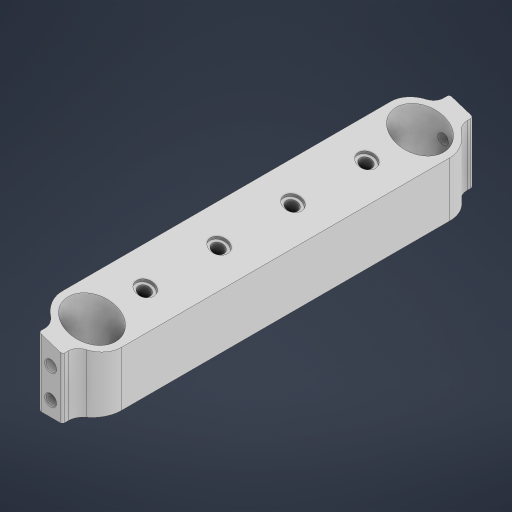
# Autodesk Inventor part: Leg_Battery_Connector
Saved by Autodesk Inventor 2023 (Build 270158000, 158)
## iProperties
Created: 2023-04-04
Part Number: Leg_Battery_Connector
Material: Generic
Document SubType Name: Modeling
Designer: dzw04
Density: 1 g/cm^3
Appearance: Default
Author: dzw04
Autodesk Inventor part; units mm, degrees
ref_plane "YZ Plane" through (0, 0, 0) normal (1, 0, 0) x (0, 1, 0)
ref_plane "XZ Plane" through (0, 0, 0) normal (0, 1, 0) x (-1, 0, 0)
ref_plane "XY Plane" through (0, 0, 0) normal (0, 0, 1) x (1, 0, 0)
sketch "Sketch1" plane through (0, 0, 0) normal (0, 1, 0) x (-1, 0, 0)
  line L0 (0, 0) -> (0, -55.5) construction
  circle A0 centre (0, -55.5) radius 8
  line L1 (0, 0) -> (10, 0) construction
  line L2 (0, 0) -> (-10, 0) construction
  line L3 (10, -55.5) -> (10, 0)
  line L4 (-10, -55.5) -> (-10, 0)
  line L5 (0, 0) -> (0, -12.5) construction
  line L6 (0, -12.5) -> (0, -37.5) construction
  line L7 (0, -65.5) -> (0, -69.5) construction
  line L8 (0, -69.5) -> (3.25, -69.5)
  line L9 (4, -68.75) -> (4, -67.5)
  line L10 (0, -69.5) -> (-3.25, -69.5)
  line L11 (-4, -68.75) -> (-4, -67.5)
  arc A1 (-10, -55.5) -> (-6, -63.5) centre (0, -55.5) ccw
  arc A2 (6, -63.5) -> (10, -55.5) centre (0, -55.5) ccw
  arc A3 (6, -63.5) -> (4, -67.5) centre (9, -67.5) ccw
  arc A4 (-4, -67.5) -> (-6, -63.5) centre (-9, -67.5) ccw
  arc A5 (-4, -68.75) -> (-3.25, -69.5) centre (-3.25, -68.75) ccw
  arc A6 (3.25, -69.5) -> (4, -68.75) centre (3.25, -68.75) ccw
  line L12 (0, 0) -> (0, 55.5) construction
  circle A7 centre (0, 55.5) radius 8
  line L13 (10, 55.5) -> (10, 0)
  line L14 (-10, 55.5) -> (-10, 0)
  line L15 (0, 0) -> (0, 12.5) construction
  line L16 (0, 12.5) -> (0, 37.5) construction
  line L17 (0, 65.5) -> (0, 69.5) construction
  line L18 (0, 69.5) -> (3.25, 69.5)
  line L19 (4, 68.75) -> (4, 67.5)
  line L20 (0, 69.5) -> (-3.25, 69.5)
  line L21 (-4, 68.75) -> (-4, 67.5)
  arc A8 (-6, 63.5) -> (-10, 55.5) centre (0, 55.5) ccw
  arc A9 (10, 55.5) -> (6, 63.5) centre (0, 55.5) ccw
  arc A10 (4, 67.5) -> (6, 63.5) centre (9, 67.5) ccw
  arc A11 (-6, 63.5) -> (-4, 67.5) centre (-9, 67.5) ccw
  arc A12 (-3.25, 69.5) -> (-4, 68.75) centre (-3.25, 68.75) ccw
  arc A13 (4, 68.75) -> (3.25, 69.5) centre (3.25, 68.75) ccw
  point P0 (4, -69.5)
  point P1 (4, -64.6652)
  point P2 (-4, -69.5)
  point P3 (-4, -64.6652)
  point P4 (4, 69.5)
  point P5 (4, 64.6652)
  point P6 (-4, 69.5)
  point P7 (-4, 64.6652)
  dimension "d0" = 55.5
  dimension "d1" = 16
  dimension "d3" = 10
  dimension "d4" = 10
  dimension "d6" = 12.5
  dimension "d7" = 25
  dimension "d10" = 4
  dimension "d11" = 4
  dimension "d12" = 4
  dimension "d13" = 5
  dimension "d14" = 0.75
  constraints: 44 end point, 28 point on circle, 25 symmetric about line, 16 point on line, 14 centre point, 10 tangent, 4 coincident, 4 horizontal, 2 equal radius, 2 perpendicular, 2 vertical, 7 other
  measures "d0" distance of L0.start L0.end
  measures "d1" diameter of A0
  measures "d3" distance of L0.start L1.end
  measures "d4" distance of L0.start L2.end
  measures "d6" distance of L0.start L5.end
  measures "d7" distance of L5.end L6.end
  measures "d10" distance of L7.start L7.end
  measures "d11" distance of L7.end point (4, -69.5)
  measures "d12" distance of L7.end point (-4, -69.5)
  measures "d13" radius of A3
  measures "d14" radius of A5
extrude "Extrusion1" add sketch "Sketch1" along normal blind 25
sketch "Sketch2" plane through (0, 0, 0) normal (0, 0, 1) x (1, 0, 0)
  line L0 (-10, 25) -> (10, 18.5016)
  line L1 (10, 0) -> (10, 25) projected
  line L2 (-10, 25) -> (11.0292, 25) construction
  line L3 (10, 18.5016) -> (10, 25)
  line L4 (10, 25) -> (-10, 25)
  point P0 (0, 0)
  dimension "d17" = 18
  constraints: 8 end point, 1 collinear, 1 equal length, 1 horizontal, 1 perpendicular, 1 point on line
  measures "d17" angle of L0 L2
extrude "Extrusion2" cut sketch "Sketch2" along normal through all both and the other way through all
sketch "Sketch3" plane through (10, 18.5016, 55.5) normal (0.309, 0.9511, 0) x (0.9511, -0.309, 0)
  ellipse E0 centre (-10.5146, 0) end of major axis (-2.1029, 0) minor radius 8 projected
  ellipse E1 centre (-10.5146, 111) end of major axis (-2.1029, 111) minor radius 8 projected
  line L0 (-10.5146, 0) -> (-10.5146, 111) construction
  line L1 (-10.5146, 55.5) -> (-10.5146, 43)
  line L2 (-10.5146, 43) -> (-10.5146, 18)
  line L3 (-10.5146, 55.5) -> (-10.5146, 68)
  line L4 (-10.5146, 68) -> (-10.5146, 93)
  circle A0 centre (-10.5146, 18) radius 2
  circle A1 centre (-10.5146, 43) radius 2
  circle A2 centre (-10.5146, 68) radius 2
  circle A3 centre (-10.5146, 93) radius 2
  point P0 (-3.7933, 55.5)
  dimension "d20" = 12.5
  dimension "d21" = 25
  dimension "d22" = 12.5
  dimension "d23" = 25
  dimension "d24" = 4
  dimension "d25" = 4
  dimension "d26" = 4
  dimension "d27" = 4
  constraints: 10 end point, 4 centre point, 4 coincident, 4 point on line, 1 midpoint, 1 vertical
  measures "d20" distance of L1.start L1.end
  measures "d21" distance of L1.end L2.end
  measures "d22" distance of L1.start L3.end
  measures "d23" distance of L3.end L4.end
  measures "d24" diameter of A0
  measures "d25" diameter of A1
  measures "d26" diameter of A2
  measures "d27" diameter of A3
extrude "Extrusion3" cut sketch "Sketch3" against normal blind 10 contours A0 | A1 L2 L1 | L1 L2 A1 | A3 | A2 L4 L3 | L3 L4 A2
sketch "Sketch4" plane through (10, 18.5016, 55.5) normal (0.309, 0.9511, 0) x (0.9511, -0.309, 0)
  circle A0 centre (-10.5146, 18) radius 2 projected
  circle A1 centre (-10.5146, 18) radius 3
  circle A2 centre (-10.5146, 43) radius 2 projected
  circle A3 centre (-10.5146, 43) radius 3
  circle A4 centre (-10.5146, 68) radius 2 projected
  circle A5 centre (-10.5146, 68) radius 3
  circle A6 centre (-10.5146, 93) radius 2 projected
  circle A7 centre (-10.5146, 93) radius 3
  point P0 (-3.7933, 55.5)
  dimension "d30" = 6
  dimension "d31" = 6
  dimension "d32" = 6
  dimension "d33" = 6
  constraints: 4 centre point, 4 coincident
  measures "d30" diameter of A1
  measures "d31" diameter of A3
  measures "d32" diameter of A5
  measures "d33" diameter of A7
extrude "Extrusion4" cut sketch "Sketch4" against normal blind 1
sketch "Sketch5" plane through (-3.25, 0, 69.5) normal (0, 0, 1) x (1, 0, 0)
  line L0 (3.25, 0) -> (3.25, 5)
  line L1 (3.25, 5) -> (3.25, 15)
  circle A0 centre (3.25, 15) radius 1.75
  circle A1 centre (3.25, 5) radius 1.75
  dimension "d36" = 5
  dimension "d37" = 10
  dimension "d38" = 3.5
  dimension "d39" = 3.5
  constraints: 4 end point, 2 centre point, 2 coincident, 1 point on line, 1 vertical
  measures "d36" distance of L0.start L0.end
  measures "d37" distance of L0.end L1.end
  measures "d38" diameter of A0
  measures "d39" diameter of A1
extrude "Extrusion5" cut sketch "Sketch5" against normal blind 7.5
sketch "Sketch6" plane through (3.25, 0, -69.5) normal (0, 0, -1) x (-1, 0, 0)
  line L0 (3.25, 0) -> (3.25, 5)
  line L1 (3.25, 5) -> (3.25, 15)
  circle A0 centre (3.25, 15) radius 1.75
  circle A1 centre (3.25, 5) radius 1.75
  dimension "d42" = 5
  dimension "d43" = 10
  dimension "d44" = 3.5
  dimension "d45" = 3.5
  constraints: 4 end point, 2 centre point, 2 coincident, 1 point on line, 1 vertical
  measures "d42" distance of L0.start L0.end
  measures "d43" distance of L0.end L1.end
  measures "d44" diameter of A0
  measures "d45" diameter of A1
extrude "Extrusion6" cut sketch "Sketch6" against normal blind 7.5
chamfer "Chamfer1" distance 0.25 angle 45 4 edges at (1.75, 5, -69.5) (1.75, 15, -69.5) (-1.75, 15, 69.5) (-1.75, 5, 69.5)
body "Solid1"
